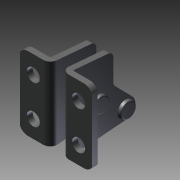
# Autodesk Inventor part: 305-U-W
Saved by Autodesk Inventor 2011 SP1 (Build 150282100, 282)
## iProperties
Created: 2018-01-28
Part Number: 305-U-W
Catalog Web Link: www.cadenas.de
Description: WF-U-KOMP-Winkelfuss
Vendor: DESTACO
Document SubType Name: Modeling
Designer: psAdmin
Manufacturer: DESTACO
Mass: 2.76401 g
Surface Area: 32.4099 cm^2
Volume: 2.76401 cm^3
Density: 1 g/cm^3
Category: PARTsolutions
Company: DESTACO
Title: 305-U-W
Author: Cadenas PARTsolutions
Comments: Winkelfuss
PSOL_IDENT_0: {$CADENAS_DATA\23d-libs\destaco\destaco_gmbh\man_spann\horizontalspanner\kompakt\u_kompakt_parts\win
PSOL_IDENT_1: kelfuss_u_komp.prj},153 {VTYP=3D},{NB=305-U-W},{LINA=305-U-W},{NN=WF-U-KOMP},{DATE=20.09.2016 07:53:
PSOL_IDENT_2: 11},{GEOMDATE=10.07.2006},{VERSION=v1},{LINEID=320},{LINESUBID=-1},{WBVAR=}  {NB=305-U-W},{LINA=305-
PSOL_IDENT_3: U-W},{KT=DUMMY},{MODELL=305-U-W},{HALTEKRAFT=650},{OEFFNUNG=90°},{GEWICHT=0.06},{ANDRUCKSPINDEL=3052
PSOL_IDENT_4: 08-M},{A=13.5},{A1=26.0},{A3=6.5},{B=16.0},{B1=25.5},{C=12.5},{C1=8.0},{C2=2},{D=4.5},{F=5.5},{H=35.
PSOL_IDENT_5: 5},{L=56.5},{L1=30.5},{L2=13.5},{L3=12.5},{M=M5},{SIZE=1},{MOD=1.000},{VER=1}
NN: WF-U-KOMP
NT: Winkelfuss
NB: 305-U-W
NBSYN: $MODELL.
LINA: 305-U-W
MODELL: 305-U-W
HALTEKRAFT: 650
OEFFNUNG: 90°
GEWICHT: 0.06
ANDRUCKSPINDEL: 305208-M
A: 13.5
A1: 26.0
A3: 6.5
B: 16.0
B1: 25.5
C: 12.5
C1: 8.0
C2: 2
D: 4.5
F: 5.5
H: 35.5
L: 56.5
L1: 30.5
L2: 13.5
L3: 12.5
M: M5
SIZE: 1
MOD: 1.000
VER: 1
SUPPLIER: DESTACO
ARTICLENO: 305-U-W
BOMINFO: 305-U-W
CREATOR: CADENAS GmbH
Autodesk Inventor part; units mm, degrees
sketch "Skizze_1" plane through (0, 0, 0) normal (0, 0, 1) x (1, 0, 0)
  arc A0 (2, 2.5) -> (4.5, 0) centre (4.5, 2.5) ccw
  line L0 (4.5, 0) -> (12.75, 0)
  line L1 (12.75, 0) -> (12.75, 2)
  line L2 (12.75, 2) -> (4.5, 2)
  arc A1 (4, 2.5) -> (4.5, 2) centre (4.5, 2.5) ccw
  line L3 (4, 2.5) -> (4, 30)
  line L4 (4, 30) -> (2, 30)
  line L5 (2, 30) -> (2, 2.5)
  constraints: 12 end point, 4 point on circle, 2 centre point
extrude "Extrusion1" add sketch "Skizze_1" along normal blind 26
sketch "Skizze_2" plane through (0, 0, 5.007) normal (0, 0, 1) x (1, 0, 0)
  line L0 (5.17, 20.6) -> (0, 20.6)
  line L1 (-5.17, 20.6) -> (-5.17, 22.89)
  arc A0 (-4.67, 23.39) -> (-5.17, 22.89) centre (-4.67, 22.89) ccw
  line L2 (-4.67, 23.39) -> (-4, 23.39)
  line L3 (-4, 23.39) -> (-4, 22.15)
  line L4 (-4, 22.15) -> (4, 22.15)
  line L5 (4, 22.15) -> (4, 23.39)
  line L6 (4, 23.39) -> (4.67, 23.39)
  arc A1 (5.17, 22.89) -> (4.67, 23.39) centre (4.67, 22.89) ccw
  line L7 (5.17, 22.89) -> (5.17, 20.6)
  line L8 (5.17, 20.6) -> (-5.17, 20.6)
  constraints: 18 end point, 4 point on circle, 2 centre point
revolve "Revolution1" add sketch "Skizze_2" angle 360 about axis through (5.17, 20.6, 5.007) along (1, 0, 0)
sketch "Skizze_3" plane through (0, 0, 11.357) normal (0, 0, 1) x (1, 0, 0)
  line L0 (5.17, 11.1) -> (0, 11.1)
  line L1 (-5.17, 11.1) -> (-5.17, 13.39)
  arc A0 (-4.67, 13.89) -> (-5.17, 13.39) centre (-4.67, 13.39) ccw
  line L2 (-4.67, 13.89) -> (-4, 13.89)
  line L3 (-4, 13.89) -> (-4, 12.65)
  line L4 (-4, 12.65) -> (4, 12.65)
  line L5 (4, 12.65) -> (4, 13.89)
  line L6 (4, 13.89) -> (4.67, 13.89)
  arc A1 (5.17, 13.39) -> (4.67, 13.89) centre (4.67, 13.39) ccw
  line L7 (5.17, 13.39) -> (5.17, 11.1)
  line L8 (5.17, 11.1) -> (-5.17, 11.1)
  constraints: 18 end point, 4 point on circle, 2 centre point
revolve "Revolution2" add sketch "Skizze_3" angle 360 about axis through (5.17, 11.1, 11.357) along (1, 0, 0)
sketch "Skizze_5" plane through (0, 0, 0) normal (0, 0, 1) x (1, 0, 0)
  line L0 (-12.75, 2) -> (-12.75, 0)
  line L1 (-12.75, 0) -> (-4.5, 0)
  arc A0 (-4.5, 0) -> (-2, 2.5) centre (-4.5, 2.5) ccw
  line L2 (-2, 2.5) -> (-2, 30)
  line L3 (-2, 30) -> (-4, 30)
  line L4 (-4, 30) -> (-4, 2.5)
  arc A1 (-4.5, 2) -> (-4, 2.5) centre (-4.5, 2.5) ccw
  line L5 (-4.5, 2) -> (-12.75, 2)
  constraints: 12 end point, 4 point on circle, 2 centre point
extrude "Extrusion2" add sketch "Skizze_5" along normal blind 26
sketch "Skizze_6" plane through (0, 0, 0) normal (1, 0, 0) x (0, 1, 0)
  line L0 (-41, 77) -> (-41, -76)
  line L1 (-41, -76) -> (70, -76)
  line L2 (70, -76) -> (70, 77)
  line L3 (70, 77) -> (-41, 77)
  line L4 (2, 26) -> (0, 26)
  line L5 (0, 26) -> (0, 0)
  line L6 (0, 0) -> (2, 0)
  line L7 (2, 0) -> (20.8805, 1.5183)
  arc A0 (20.8805, 1.5183) -> (23.1011, 7.4554) centre (20.6, 5.007) ccw
  line L8 (23.1011, 7.4554) -> (16.8708, 13.8197)
  arc A1 (16.3, 15.2188) -> (16.8708, 13.8197) centre (18.3, 15.2188) ccw
  line L9 (16.3, 15.2188) -> (16.3, 22.9162)
  arc A2 (16.3, 22.9162) -> (14.4743, 24.9086) centre (14.3, 22.9162) ccw
  line L10 (14.4743, 24.9086) -> (2, 26)
  constraints: 22 end point, 6 point on circle, 3 centre point
extrude "Extrusion3" cut sketch "Skizze_6" along normal mid plane 100
sketch "Skizze_7" plane through (0, 0, 0) normal (0, 1, 0) x (-1, 0, 0)
  line L0 (50, 50) -> (-61, 50)
  line L1 (-61, 50) -> (-61, -33)
  line L2 (-61, -33) -> (50, -33)
  line L3 (50, -33) -> (50, 50)
  arc A0 (13, 23) -> (10, 26) centre (10, 23) ccw
  line L4 (10, 26) -> (-10, 26)
  arc A1 (-10, 26) -> (-13, 23) centre (-10, 23) ccw
  line L5 (-13, 23) -> (-13, 3)
  arc A2 (-13, 3) -> (-10, 0) centre (-10, 3) ccw
  line L6 (-10, 0) -> (10, 0)
  arc A3 (10, 0) -> (13, 3) centre (10, 3) ccw
  line L7 (13, 3) -> (13, 23)
  constraints: 16 end point, 8 point on circle, 4 centre point
extrude "Extrusion4" cut sketch "Skizze_7" along normal blind 2
sketch "Skizze_8_ALT_Drilling_1" plane through (0, 0, 0) normal (0, 1, 0) x (-1, 0, 0)
  circle A0 centre (-8, 6.15) radius 2.3
  constraints: 1 centre point
extrude "Extrusion5" cut sketch "Skizze_8_ALT_Drilling_1" along normal blind 2
sketch "Skizze_9_ALT_Drilling_2" plane through (0, 0, 0) normal (0, 1, 0) x (-1, 0, 0)
  circle A0 centre (-8, 19.65) radius 2.3
  constraints: 1 centre point
extrude "Extrusion6" cut sketch "Skizze_9_ALT_Drilling_2" along normal blind 2
sketch "Skizze_10_ALT_Drilling_3" plane through (0, 0, 0) normal (0, 1, 0) x (-1, 0, 0)
  circle A0 centre (8, 6.15) radius 2.3
  constraints: 1 centre point
extrude "Extrusion7" cut sketch "Skizze_10_ALT_Drilling_3" along normal blind 2
sketch "Skizze_11_ALT_Drilling_4" plane through (0, 0, 0) normal (0, 1, 0) x (-1, 0, 0)
  circle A0 centre (8, 19.65) radius 2.3
  constraints: 1 centre point
extrude "Extrusion8" cut sketch "Skizze_11_ALT_Drilling_4" along normal blind 2
ref_plane "WF1_XY" through (0, 20.6, 5.007) normal (1, 0, 0) x (0, 0, -1)
ref_plane "WF1_YZ" through (0, 20.6, 5.007) normal (0, 0, -1) x (0, 1, 0)
ref_plane "WF1_ZX" through (0, 20.6, 5.007) normal (0, 1, 0) x (1, 0, 0)
ref_plane "WF2_XY" through (0, 11.1, 11.357) normal (1, 0, 0) x (0, 0, -1)
ref_plane "WF2_YZ" through (0, 11.1, 11.357) normal (0, 0, -1) x (0, 1, 0)
ref_plane "WF2_ZX" through (0, 11.1, 11.357) normal (0, 1, 0) x (1, 0, 0)
body "Solid1"
